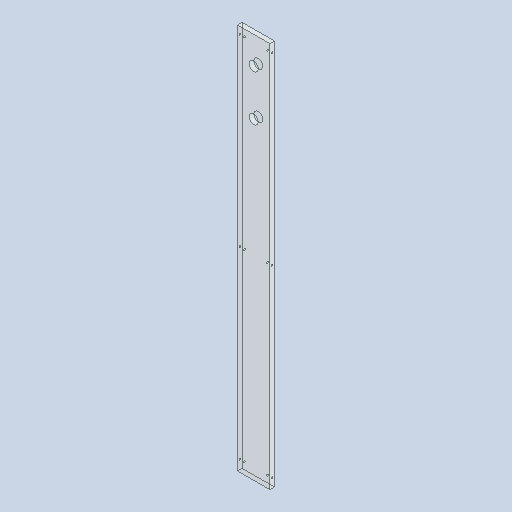
# Autodesk Inventor part: Side plate profile
Saved by Autodesk Inventor 2022 (Build 260153000, 153)
## iProperties
Created: 2021-11-04
Part Number: Side plate profile
Material: Acetalharz, Weiß
Document SubType Name: Modeling
Designer: espen
Density: 1.425 g/cm^3
Appearance: Klar
Mass: 103.484 g
Surface Area: 341.385 cm^2
Volume: 72.6204 cm^3
Author: espen
Autodesk Inventor part; units mm, degrees
ref_plane "YZ Plane" through (0, 0, 0) normal (1, 0, 0) x (0, 1, 0)
ref_plane "XZ Plane" through (0, 0, 0) normal (0, 1, 0) x (-1, 0, 0)
ref_plane "XY Plane" through (0, 0, 0) normal (0, 0, 1) x (1, 0, 0)
sketch "Sketch1" plane through (0, 0, 0) normal (0, 0, 1) x (1, 0, 0)
  line L0 (0, 0) -> (35, 0)
  line L1 (35, 0) -> (35, 420)
  line L2 (35, 420) -> (0, 420)
  line L3 (0, 420) -> (0, 0)
  dimension "d0" = 35
  dimension "d1" = 420
  constraints: 8 end point, 2 parallel, 1 horizontal, 1 perpendicular
  measures "d0" distance of L0.start L0.end
  measures "d1" distance of L0.end L1.end
extrude "Extrusion1" add sketch "Sketch1" along normal blind 5
sketch "Sketch2" plane through (35, 0, 0) normal (1, 0, 0) x (0, 0, -1)
  circle A0 centre (-2.5, 410) radius 1
  circle A1 centre (-2.5, 210) radius 1
  circle A2 centre (-2.5, 10) radius 1
  line L0 (-5, 0) -> (-5, 420) projected
  line L1 (0, 420) -> (-5, 420) projected
  point P0 (0, 0)
  dimension "d4" = 2
  dimension "d5" = 2
  dimension "d6" = 2
  dimension "d7" = 2.5
  dimension "d8" = 2.5
  dimension "d9" = 2.5
  dimension "d10" = 10
  dimension "d11" = 210
  dimension "d12" = 410
  constraints: 3 centre point
  measures "d4" diameter of A2
  measures "d5" diameter of A1
  measures "d6" diameter of A0
  measures "d7" distance from line of A2.centre L0
  measures "d8" distance from line of L0 A1.centre
  measures "d9" distance from line of L0 A0.centre
  measures "d10" distance from line of L1 A0.centre
  measures "d11" distance from line of L1 A1.centre
  measures "d12" distance from line of L1 A2.centre
extrude "Extrusion2" cut sketch "Sketch2" against normal blind 5
sketch "Sketch3" plane through (0, 0, 0) normal (-1, 0, 0) x (0, 0, 1)
  circle A0 centre (2.5, 10) radius 1
  circle A1 centre (2.5, 210) radius 1
  circle A2 centre (2.5, 410) radius 1
  line L0 (0, 420) -> (0, 0) projected
  line L1 (0, 420) -> (5, 420) projected
  dimension "d15" = 2
  dimension "d16" = 2.5
  dimension "d17" = 10
  dimension "d18" = 2
  dimension "d19" = 2.5
  dimension "d20" = 210
  dimension "d21" = 2
  dimension "d22" = 2.5
  dimension "d23" = 410
  constraints: 3 centre point
  measures "d15" diameter of A2
  measures "d16" distance from line of L0 A2.centre
  measures "d17" distance from line of A2.centre L1
  measures "d18" diameter of A1
  measures "d19" distance from line of L0 A1.centre
  measures "d20" distance from line of L1 A1.centre
  measures "d21" diameter of A0
  measures "d22" distance from line of L0 A0.centre
  measures "d23" distance from line of L1 A0.centre
extrude "Extrusion3" cut sketch "Sketch3" against normal blind 5
sketch "Skizze4" plane through (0, 0, 5) normal (0, 0, 1) x (1, 0, 0)
  circle A0 centre (17.5, 340) radius 5
  circle A1 centre (17.5, 390) radius 5
  line L0 (0, 420) -> (0, 0) projected
  line L1 (0, 0) -> (35, 0) projected
  line L2 (35, 420) -> (0, 420) projected
  line L3 (17.5, 420) -> (17.5, 340) construction
  dimension "d26" = 17.5
  dimension "d27" = 17.5
  dimension "d29" = 50
  dimension "d32" = 30
  dimension "d33" = 10
  constraints: 2 centre point, 2 end point, 1 equal radius, 1 midpoint
  measures "d26" distance from line of L0 L3.end
  measures "d27" distance from line of L0 A1.centre
  measures "d29" distance of L3.end A1.centre
  measures "d32" distance from line of A1.centre L2
  measures "d33" diameter of A1
extrude "Extrusion4" cut sketch "Skizze4" against normal blind 35
equation "\"d29\" = ParallelMech_LINK_GabelDist"
equation "\"d30\" = d28"
equation "\"ParallelMech_LINK_GabelDist\" = 50"
equation "\"d28\" = 35"
body "Solid1"
